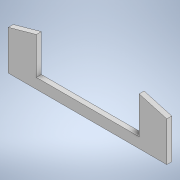
# Autodesk Inventor part: frontOfHouse
Saved by Autodesk Inventor 2020.1 (Build 241239000, 239)
## iProperties
Created: 2019-08-10
Part Number: frontOfHouse
Material: Generic
Document SubType Name: Modeling
Designer: steele
Density: 1 g/cm^3
Appearance: Default
Author: steele
Autodesk Inventor part; units mm, degrees
ref_plane "YZ Plane" through (0, 0, 0) normal (1, 0, 0) x (0, 1, 0)
ref_plane "XZ Plane" through (0, 0, 0) normal (0, 1, 0) x (-1, 0, 0)
ref_plane "XY Plane" through (0, 0, 0) normal (0, 0, 1) x (1, 0, 0)
sketch "Sketch1" plane through (0, 0, 0) normal (0, 0, 1) x (1, 0, 0)
  line L0 (0, 0) -> (-4876.8, 0)
  line L1 (-4876.8, 0) -> (-4876.8, 2438.4)
  line L2 (0, 635) -> (0, 5709.6647) construction
  line L3 (-3149.6, 635) -> (-3149.6, 2921)
  line L4 (0, 0) -> (0, 635)
  line L5 (0, 635) -> (-3149.6, 635)
  line L6 (-4876.8, 2438.4) -> (-3149.6, 2921)
  line L7 (0, 0) -> (4876.8, 0)
  line L8 (4876.8, 0) -> (4876.8, 2438.4)
  line L9 (4876.8, 2438.4) -> (3175, 2921)
  line L10 (0, 635) -> (3175, 635)
  line L11 (3175, 635) -> (3175, 2921)
  dimension "d0" = 4876.8
  dimension "d1" = 2438.4
  dimension "d3" = 1727.2
  dimension "d4" = 635
  dimension "d5" = 2921
  dimension "d6" = 4876.8
  dimension "d7" = 2438.4
  dimension "d8" = 2921
  dimension "d11" = 9753.6
  dimension "d12" = 1701.8
  dimension "d13" = 2286
  dimension "d14" = 2286
  dimension "d15" = 1793.3551
  dimension "d16" = 1768.9053
  dimension "d17" = 6324.6
  dimension "d18" = 3149.6
  dimension "d19" = 3175
  constraints: 24 end point, 3 horizontal, 3 perpendicular, 3 vertical
  measures "d0" distance of L0.start L0.end
  measures "d1" distance of L0.end L1.end
  measures "d3" distance between parallel lines of L3 L1
  measures "d4" distance of L2.start L0.start
  measures "d5" distance from line of L3.end L0
  measures "d6" distance of L0.start L7.end
  measures "d7" distance of L7.end L8.end
  measures "d8" distance from line of L9.end L7
  measures "d11" distance between parallel lines of L1 L8
  measures "d12" distance between parallel lines of L8 L11
  measures "d13" distance of L3.end L3.start
  measures "d14" distance of L9.end L10.end
  measures "d15" distance of L3.end L1.end
  measures "d16" distance of L8.end L9.end
  measures "d17" distance of L10.end L3.start
  measures "d18" distance of L2.start L3.start
  measures "d19" distance of L10.end L2.start
extrude "Extrusion1" add sketch "Sketch1" against normal blind 304.8
body "Solid1"
